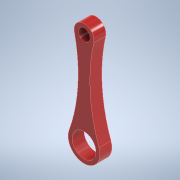
# Autodesk Inventor part: Connecting_Rod
Saved by Autodesk Inventor 2021 (Build 250183000, 183)
## iProperties
Created: 2021-04-09
Part Number: Connecting_Rod
Material: Titanium
Document SubType Name: Modeling
Designer: tommy
Density: 4.51 g/cm^3
Appearance: Red
bore_dia: 4.000 in
piston_height: 3.000 in
d3: 0.00 deg
wall_thick: 0.250 in
d6: 2.750 in
d7: 0.00 deg
pin_dia: 0.750 in
d11: 1.500 in
d12: 0.750 in
d14: 0.00 deg
ring_depth: 0.100 in
ring_height: 0.150 in
ring_offset: 0.250 in
d19: 3.000 ul
ring_spacing: 0.300 in
Author: tommy
Autodesk Inventor part; units mm, degrees
ref_plane "YZ Plane" through (0, 0, 0) normal (1, 0, 0) x (0, 1, 0)
ref_plane "XZ Plane" through (0, 0, 0) normal (0, 1, 0) x (-1, 0, 0)
ref_plane "XY Plane" through (0, 0, 0) normal (0, 0, 1) x (1, 0, 0)
sketch "Sketch1" plane through (0, 0, 0) normal (0, 0, 1) x (1, 0, 0)
  circle A0 centre (0, 0) radius 9.525
  circle A1 centre (0, -152.4) radius 19.05
  line L0 (0, -216.535) -> (0, 54.61) construction
  circle A2 centre (0, 0) radius 15.875
  circle A3 centre (0, -152.4) radius 25.4
  arc A4 (-23.9399, -143.9123) -> (-15.4905, -3.4727) centre (-263.3389, -59.0352) ccw
  arc A5 (15.4905, -3.4727) -> (23.9399, -143.9123) centre (263.3389, -59.0352) ccw
  point P0 (23.9399, -143.9123)
  point P1 (15.4905, -3.4727)
  dimension "d0" = 19.05
  dimension "d1" = 38.1
  dimension "conrod_ctc" = 152.4
  dimension "conrod_wt" = 6.35
  dimension "d5" = 6.35
  dimension "conrod_rad" = 254
  constraints: 4 centre point, 4 point on circle, 3 symmetric about line, 2 coincident, 1 point on line, 9 other
  measures "d0" diameter of A0
  measures "d1" diameter of A1
  measures "conrod_ctc" distance of point (0, 0) A1.centre
  measures "conrod_rad" radius of A4
extrude "Extrusion1" add sketch "Sketch1" along normal mid plane 19.05
equation "\"d0\" = pin_dia"
equation "\"d1\" = 2 * d0"
equation "\"d5\" = conrod_wt"
equation "\"pin_dia\" = 19.05"
body "Solid1"
